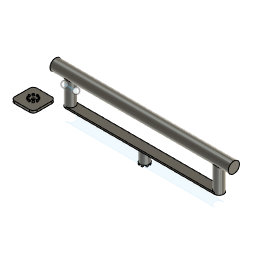
Pulls1 v5 (Autodesk Fusion 360 design; units mm, degrees)
Autodesk Fusion 360 part; units mm, degrees
note: some values were not read from the file. Chosen so that the rebuilt part matches the saved one: which bodies a step acts on. Set by a fixed rule: which sketch regions a step uses.
sketch "Sketch1" plane through (0, 0, 0) normal (0, 0, 1) x (1, 0, 0)
  circle A0 centre (0, 0) radius 6.25
  dimension "d1" = 12.5
  constraint coincident A0.centre origin
  measures "d1" diameter of A0
extrude "Extrude1" add sketch "Sketch1" along normal blind 2 makes body 1
copy_body "Body->Comp1" bodies 1 removing the originals makes body 2 in component "Teeth"
sketch "Sketch2" plane through (0, 0, 2) normal (0, 0, 1) x (-1, 0, 0)
  circle A0 centre (0, 0) radius 6.25
  line L0 (0, 0) -> (0, -7)
  line L1 (0, 0) -> (2.6788, -6.4672)
  line L2 (0, 0) -> (4.9497, -4.9497)
  line L3 (0, 0) -> (6.4672, -2.6788)
  line L4 (0, 0) -> (7, 0)
  line L5 (0, 0) -> (6.4672, 2.6788)
  line L6 (0, 0) -> (4.9497, 4.9497)
  line L7 (0, 0) -> (2.6788, 6.4672)
  line L8 (0, 0) -> (0, 7)
  line L9 (0, 0) -> (-2.6788, 6.4672)
  line L10 (0, 0) -> (-4.9497, 4.9497)
  line L11 (0, 0) -> (-6.4672, 2.6788)
  line L12 (0, 0) -> (-7, 0)
  line L13 (0, 0) -> (-6.4672, -2.6788)
  line L14 (0, 0) -> (-4.9497, -4.9497)
  line L15 (0, 0) -> (-2.6788, -6.4672)
  dimension "d5" = 360
  constraint coincident A0.centre L0.start
  constraint vertical L0
split "Split1" by curves path "Sketch2" along L15 L0 bodies 2 makes body 3 at (2.8653, -3.0095, 0) in component "Teeth"
move_body "Move1" bodies 2 to x (0.980785, 0.19509, 0) y (-0.19509, 0.980785, 0) z (0, 0, 1) at (0, 0, 0) in component "Teeth"
hole "Hole1" at (0, 0, 2) direction (0, 0, -1) diameter 10 depth 6 tip angle 118 bodies 2 in component "Teeth"
fillet "Fillet1" radius 0.5 2 edges at (-1.0974, 5.5169, 2) (1.0974, 5.5169, 2) on bodies 2 in component "Teeth"
pattern_circular "C-Pattern1" count 8 over 360 about axis through (0, 0, 1.75) along (0, 0, 1) of bodies 2 makes body 4 at (-4.8393, 3.9552, 1.1667) makes body 5 at (-6.2187, 0.6251, 1.1667) makes body 6 at (-3.9552, -4.8393, 1.1667) makes body 7 at (-0.6251, -6.2187, 1.1667) makes body 8 at (4.8393, -3.9552, 1.1667) makes body 9 at (6.2187, -0.6251, 1.1667) makes body 10 at (3.9552, 4.8393, 1.1667) in component "Teeth"
sketch "Sketch1 (2)" plane through (0, 0, 0) normal (0, 0, 1) x (1, 0, 0) in component "Backplate"
  line L0 (-15, 15) -> (15, 15)
  line L1 (15, 15) -> (15, -15)
  line L2 (15, -15) -> (-15, -15)
  line L3 (-15, -15) -> (-15, 15)
  constraint horizontal L0
  constraint vertical L1
  constraint horizontal L2
  constraint vertical L3
extrude "Extrude1'" add sketch "Sketch1 (2)" along normal blind 3 separate body makes body 11 in component "Backplate"
fillet "Fillet1'" radius 5 4 edges at (-15, -15, 1.5) (15, -15, 1.5) (-15, 15, 1.5) (15, 15, 1.5) on bodies 11 in component "Backplate"
hole "Hole1'" at (0, 0, 3) direction (0, 0, -1) diameter 3.75 depth 6 tip angle 118 bodies 11 in component "Backplate"
hole "Hole2" at (0, 0, 0) direction (0, 0, 1) diameter 3.75 depth 16 tip angle 118 countersink diameter 5 countersink angle 45 bodies 11 in component "Backplate"
combine "Combine1" operation add target body 11 tool bodies 2 4 5 body 2 seen with x (1, 0, 0) y (0, 1, 0) z (0, 0, 1) at (0, 0, 3) body 4 seen with x (1, 0, 0) y (0, 1, 0) z (0, 0, 1) at (0, 0, 3) body 5 seen with x (1, 0, 0) y (0, 1, 0) z (0, 0, 1) at (0, 0, 3) in component "Backplate"
combine "Combine1'" operation add target body 6 tool bodies 9 8 7 10 11 body 11 seen with x (1, 0, 0) y (0, 1, 0) z (0, 0, 1) at (0, 0, -3) in component "Teeth"
sketch "Sketch2 (2)" plane through (0, 0, 0) normal (0, 0, 1) x (1, 0, 0) in component "Backplate"
sketch "Sketch1 (3)" plane through (0, 0, 0) normal (0, 1, 0) x (1, 0, 0) in component "BarHandle"
sketch "Sketch2 (3)" plane through (0, 0, 0) normal (0, 0, 1) x (1, 0, 0) in component "BarHandle"
  circle A0 centre (50, 0) radius 6.25
  circle A1 centre (250, 0) radius 6.25
  dimension "d26" = 12.5
  dimension "d27" = 12.5
  measures "d26" diameter of A0
  measures "d27" diameter of A1
extrude "Extrude1''" add sketch "Sketch2 (3)" along normal blind 38.25 separate body makes body 12 at (56.2422, -0.3115, 25.5) makes body 13 at (251.0853, 6.155, 25.5) in component "BarHandle"
sketch "Sketch3" plane through (0, 0, 0) normal (0, 0, -1) x (1, 0, 0) in component "BarHandle"
  circle A0 centre (50, 0) radius 6.25
  line L0 (50, 7.5) -> (50, -7.5) construction
  line L1 (250, -10) -> (250, 10) construction
  line L2 (250, 10) -> (254, 11) construction
  line L3 (50, 6.25) -> (250, 6.25)
  line L4 (250, 6.25) -> (250, -6.25)
  line L5 (250, -6.25) -> (50, -6.25)
  line L6 (50, -6.25) -> (50, 6.25)
  constraint vertical L0
  constraint parallel L0 L1
  constraint horizontal L3
  constraint vertical L4
  constraint horizontal L5
  constraint vertical L6
  constraint coincident L1 L4.end
  constraint coincident L0 L3.start
  constraint coincident A0 L3.start
extrude "Extrude2" add sketch "Sketch3" against normal blind 2 contours A0 L3 L4 L5 bodies 13 12 in component "BarHandle"
sketch "Sketch4" plane through (0, 0, 2) normal (0, 0, 1) x (-1, 0, 0) in component "BarHandle"
  arc A0 (-250, -6.25) -> (-250, 6.25) centre (-250, 0) ccw
  line L0 (-250, -6.25) -> (-50, -6.25)
  arc A1 (-50, 6.25) -> (-50, -6.25) centre (-50, 0) ccw
  line L1 (-50, 6.25) -> (-250, 6.25)
sketch "Sketch5" plane through (0, 0, 38.25) normal (0, 0, 1) x (-1, 0, 0) in component "BarHandle"
  circle A0 centre (-50, 0) radius 6.25
  line L0 (-42.5, 0) -> (-57.5, 0)
  constraint horizontal L0
sketch "Sketch6" plane through (0, 0, 0) normal (1, 0, 0) x (0, 1, 0) in component "BarHandle"
  line L0 (7.5, 38) -> (-7, 38)
  line L1 (-7, 38) -> (-7.5, 38)
  circle A0 centre (0, 38.25) radius 7.5
  dimension "d32" = 15
  constraint horizontal L0
  constraint parallel L0 L1
  measures "d32" diameter of A0
extrude "Extrude3" add sketch "Sketch6" along normal blind 210 separate body makes body 14 in component "BarHandle"
move_body "Move1'" bodies 14 to x (1, 0, 0) y (0, 1, 0) z (0, 0, 1) at (60, 0, 0) in component "BarHandle"
extrude "Extrude4" add 1 faces at (60, -2.2688, 40.1588) along direction (-1, 0, 0) blind 30 on bodies 14 bodies 14 13 in component "BarHandle"
sketch "Sketch7" plane through (0, 0, 0) normal (0, 0, -1) x (1, 0, 0) in component "BarHandle"
  arc A0 (250, -6.25) -> (250, 6.25) centre (250, 0) ccw
  line L0 (250, 6.25) -> (50, 6.25)
  arc A1 (50, 6.25) -> (50, -6.25) centre (50, 0) ccw
  line L1 (50, -6.25) -> (250, -6.25)
  line L2 (52.4535, 6.25) -> (52.4535, -6.25) construction
  line L3 (43.75, 0) -> (256.25, 0) construction
  circle A2 centre (150, 0) radius 6.25
  dimension "d40" = 12.5
  constraint coincident L0 L2.start
  constraint coincident L1 L2.end
  constraint perpendicular L1 L2
  constraint midpoint A1 L3.start
  constraint midpoint A0 L3.end
  constraint midpoint L3 A2.centre
  measures "d40" diameter of A2
extrude "Extrude5" add sketch "Sketch7" along normal blind 15 contours A2 bodies 14 in component "BarHandle"
copy_body "CopyPasteBodies1" bodies 6 6 6 6 6 6 6 6 makes body 15 in component "BarHandle"
move_body "Move2" bodies 15 to x (1, 0, 0) y (0, 1, 0) z (0, 0, 1) at (150, 0, -20) in component "BarHandle"
sketch "Sketch3 (2)" plane through (0, -15, 0) normal (0, -1, 0) x (1, 0, 0)
  line L0 (160, -23) -> (160, -20)
  line L1 (160, -20) -> (140, -20)
  line L2 (140, -20) -> (140, -23)
  line L3 (140, -23) -> (160, -23)
  line L4 (132, -20) -> (168, -20)
  line L5 (168, -20) -> (168, -25)
  line L6 (168, -25) -> (132, -25)
  line L7 (132, -25) -> (132, -20)
  constraint horizontal L4
  constraint vertical L5
  constraint horizontal L6
  constraint vertical L7
extrude "Extrude6" cut sketch "Sketch3 (2)" against normal blind 40 bodies 15 makes body 16 at (143.7813, 0.6251, -18.8333) makes body 17 at (146.0448, 4.8393, -18.8333) makes body 18 at (150.6251, 6.2187, -18.8333) makes body 19 at (153.9552, 4.8393, -18.8333) makes body 20 at (153.9552, -4.8393, -18.8333) makes body 21 at (146.0448, -4.8393, -18.8333) makes body 22 at (156.2187, -0.6251, -18.8333) in component "BarHandle"
move_body "Move3" bodies 22 19 20 15 21 16 17 18 to x (1, 0, 0) y (0, -1, 0) z (0, 0, -1) at (0, 12.5, 0) in component "BarHandle"
move_body "Move4" bodies 17 20 18 22 21 15 16 19 to x (1, 0, 0) y (0, 1, 0) z (0, 0, 1) at (0, -12.5, -35) in component "BarHandle"
sketch "Sketch4 (2)" plane through (0, 0, 2) normal (0, 0, 1) x (-1, 0, 0)
  line L0 (-143.75, 0) -> (-156.25, 0) construction
  line L1 (-150, 0) -> (-150.8484, 0)
  line L2 (-150.8484, 0) -> (-150.8484, -0.8718)
  line L3 (-150.8484, -0.8718) -> (-150, -0.8718)
  line L4 (-150, -0.8718) -> (-150, 0)
  constraint horizontal L0
  constraint horizontal L1
  constraint vertical L2
  constraint horizontal L3
  constraint vertical L4
  constraint midpoint L0 L1.start
extrude "Extrude7" add sketch "Sketch4 (2)" along normal blind 0.5 bodies 14 in component "BarHandle"
move_body "Move5" bodies 17 18 19 22 20 15 21 16 to x (0.906308, 0.422618, 0) y (-0.422618, 0.906308, 0) z (0, 0, 1) at (14.0538, -63.3927, 0) in component "BarHandle"
move_body "Move6" bodies 16 18 19 22 20 15 21 17 to x (0.67559, -0.737277, 0) y (0.737277, 0.67559, 0) z (0, 0, 1) at (48.6615, 110.5916, 0) in component "BarHandle"
sketch "Sketch5 (2)" plane through (0, 0, 0) normal (0, -1, 0) x (1, 0, 0)
  line L0 (150, 2) -> (150.8484, 2)
  line L1 (150.8484, 2) -> (150.8484, 2.5)
  line L2 (150.8484, 2.5) -> (150, 2.5)
  line L3 (150, 2.5) -> (150, 2)
  line L4 (150, 2.5) -> (150.8484, 2.5)
  line L5 (150.8484, 2.5) -> (150.8484, 2)
  line L6 (150.8484, 2) -> (150, 2)
  line L7 (150, 2) -> (150, 2.5)
  constraint horizontal L4
  constraint vertical L5
  constraint horizontal L6
  constraint vertical L7
  constraint coincident L0.end L1.start
  constraint coincident L2.end L3.start
extrude "Extrude8" cut sketch "Sketch5 (2)" against normal blind 1.05 bodies 14 in component "BarHandle"
combine "Combine1''" operation add target body 14 tool bodies 17 18 19 22 20 15 21 16 in component "BarHandle"
move_body "Move7" bodies 14 to x (1, 0, 0) y (0, 1, 0) z (0, 0, 1) at (0, 0, 17) in component "BarHandle"
component "Teeth" placed x (1, 0, 0) y (0, 1, 0) z (0, 0, 1) at (0, 0, 0)
component "Backplate" placed x (1, 0, 0) y (0, 1, 0) z (0, 0, 1) at (0, 0, 0)
component "BarHandle" placed x (1, 0, 0) y (0, 1, 0) z (0, 0, 1) at (0, 0, 0)
component "Teeth" placed x (1, 0, 0) y (0, 1, 0) z (0, 0, 1) at (0, 0, 3) in component "Backplate"
hidden bodies 3
